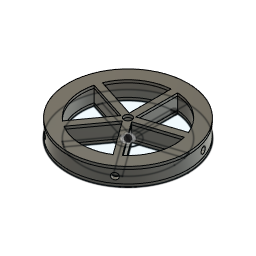
RotarySubAssembly (Autodesk Fusion 360 archive; units mm, degrees)
design "RotarySubFixedTopperV2"
Autodesk Fusion 360 part; units mm, degrees
sketch "Sketch1" plane through (0, 0, 0) normal (0, 1, 0) x (1, 0, 0)
  circle A0 centre (0, 0) radius 3
  circle A1 centre (0, 0) radius 8
  line L0 (0, 0) -> (0, 35)
  line L1 (0, 35) -> (-2.5, 35)
  line L2 (0, 35) -> (2.5, 35)
  line L3 (-2.5, 35) -> (-2.5, 0.0004)
  line L4 (-2.5, 0.0004) -> (2.5, 0.0004)
  line L5 (2.5, 0.0004) -> (2.5, 35)
  line L6 (0.7721, 2.3778) -> (-32.5144, 13.1932)
  line L7 (-34.0595, 8.438) -> (-0.773, -2.3775)
  line L8 (-33.287, 10.8156) -> (-34.0595, 8.438)
  line L9 (-33.287, 10.8156) -> (-32.5144, 13.1932)
  line L10 (-2.0228, 1.4691) -> (-22.595, -26.8461)
  line L11 (-18.5499, -29.7851) -> (2.0223, -1.4698)
  line L12 (-20.5725, -28.3156) -> (-18.5499, -29.7851)
  line L13 (-20.5725, -28.3156) -> (-22.595, -26.8461)
  line L14 (-2.0223, -1.4698) -> (18.5499, -29.7851)
  line L15 (22.595, -26.8461) -> (2.0228, 1.4691)
  line L16 (20.5725, -28.3156) -> (22.595, -26.8461)
  line L17 (20.5725, -28.3156) -> (18.5499, -29.7851)
  line L18 (0.773, -2.3775) -> (34.0595, 8.438)
  line L19 (32.5144, 13.1932) -> (-0.7721, 2.3778)
  line L20 (33.287, 10.8156) -> (32.5144, 13.1932)
  line L21 (33.287, 10.8156) -> (34.0595, 8.438)
  circle A2 centre (0, 0) radius 35
  line L22 (0, 35) -> (0, 45)
  circle A3 centre (0, 0) radius 45
  point P0 (0, 35)
  dimension "d1" = 6
  dimension "d2" = 16
  dimension "d3" = 35
  dimension "d4" = 2.5
  dimension "d6" = 360
  dimension "d7" = 10
  constraint coincident A0.centre A1.centre
  constraint vertical L0
  constraint perpendicular L0 L1
  constraint perpendicular L0 L2
  constraint equal L1 L2
  constraint perpendicular L1 L3
  constraint perpendicular L3 L4
  constraint perpendicular L2 L5
  constraint concentric A0 A2
  constraint coincident P0 L0.end
  constraint tangent L2 A2
  constraint perpendicular L1 L22
  constraint concentric A1 A3
  constraint coincident L22.end A3
  measures "d1" diameter of A0
  measures "d2" diameter of A1
  measures "d3" distance of A0.centre P0
  measures "d4" distance of P0 L1.end
  measures "d7" distance of P0 L22.end
extrude "Extrude1" add sketch "Sketch1" along normal blind 2 contours A0 L15 L18 | A0 A1 L5 L15 L18 L19 | A0 A1 L11 L14 L15 L18 | A0 L5 L19 | A0 L11 L14 | A0 A1 L0 L5 L19 | A1 L14 L15 A2 | A1 L18 L19 A2 | A0 A1 L7 L10 L11 L14 | A0 A1 L0 L3 L6 | A1 L0 L5 A2 | L15 L16 A2 | L18 L21 A2 | A0 L7 L10 | A1 L10 L11 A2 | A0 L3 L6 | A1 L0 L3 A2 | L2 L5 A2 | L19 L20 A2 | L14 L17 A2 | A0 A1 L3 L6 L7 L10 | L11 L12 A2 | L1 L3 A2 | A1 L6 L7 A2 | L10 L13 A2 | L7 L8 A2 | L6 L9 A2 | A3 makes body 1
sketch "Sketch2" plane through (0, 2, 0) normal (0, 1, 0) x (-1, 0, 0)
  arc A0 (-32.4294, -13.1656) -> (-2.5, -34.9106) centre (0, 0) ccw
  line L0 (-32.4294, -13.1656) -> (-2.5, -3.441)
  line L1 (-2.5, -3.441) -> (-2.5, -34.9106)
  arc A1 (2.5, -34.9106) -> (32.4294, -13.1656) centre (0, 0) ccw
  line L2 (2.5, -34.9106) -> (2.5, -3.441)
  line L3 (2.5, -3.441) -> (32.4294, -13.1656)
  line L4 (-22.5425, 26.7738) -> (-4.0451, 1.3143)
  line L5 (-4.0451, 1.3143) -> (-33.9745, -8.4103)
  arc A2 (-22.5425, 26.7738) -> (-33.9745, -8.4103) centre (0, 0) ccw
  arc A3 (33.9745, -8.4103) -> (22.5425, 26.7738) centre (0, 0) ccw
  line L6 (33.9745, -8.4103) -> (4.0451, 1.3143)
  line L7 (4.0451, 1.3143) -> (22.5425, 26.7738)
  arc A4 (18.4974, 29.7127) -> (-18.4974, 29.7127) centre (0, 0) ccw
  line L8 (18.4974, 29.7127) -> (0, 4.2533)
  line L9 (0, 4.2533) -> (-18.4974, 29.7127)
  circle A5 centre (0, 0) radius 3
  circle A6 centre (0, 0) radius 45
  circle A7 centre (0, 0) radius 35
  circle A8 centre (0, 0) radius 45
  line L10 (4.75, -41.9) -> (-4.75, -41.9)
  line L11 (-4.75, -41.9) -> (-4.75, -38.1)
  line L12 (-4.75, -38.1) -> (4.75, -38.1)
  line L13 (4.75, -38.1) -> (4.75, -41.9)
  line L14 (0, -35) -> (0, -38.1)
  line L15 (0, -45) -> (0, -41.9)
  line L16 (41.3171, -8.4303) -> (38.3814, -17.4653)
  line L17 (38.3814, -17.4653) -> (34.7674, -16.2911)
  line L18 (37.7031, -7.256) -> (41.3171, -8.4303)
  line L19 (34.7674, -16.2911) -> (37.7031, -7.256)
  line L20 (20.7854, 36.6898) -> (28.471, 31.1058)
  line L21 (28.471, 31.1058) -> (26.2374, 28.0316)
  line L22 (18.5518, 33.6155) -> (20.7854, 36.6898)
  line L23 (26.2374, 28.0316) -> (18.5518, 33.6155)
  line L24 (-28.471, 31.1058) -> (-20.7854, 36.6898)
  line L25 (-20.7854, 36.6898) -> (-18.5518, 33.6155)
  line L26 (-26.2374, 28.0316) -> (-28.471, 31.1058)
  line L27 (-18.5518, 33.6155) -> (-26.2374, 28.0316)
  line L28 (-38.3814, -17.4653) -> (-41.3171, -8.4303)
  line L29 (-41.3171, -8.4303) -> (-37.7031, -7.256)
  line L30 (-34.7674, -16.2911) -> (-38.3814, -17.4653)
  line L31 (-37.7031, -7.256) -> (-34.7674, -16.2911)
  dimension "d10" = 9.5
  dimension "d11" = 3.8
  dimension "d13" = 360
  constraint horizontal L10
  constraint vertical L11
  constraint horizontal L12
  constraint vertical L13
  constraint coincident A7 L14.start
  constraint vertical L14
  constraint midpoint L12 L14.end
  constraint coincident A6 L15.start
  constraint vertical L15
  constraint midpoint L10 L15.end
  constraint equal L14 L15
  constraint vertical A0.centre L14.end
  measures "d10" distance of L10.start L10.end
  measures "d11" distance of L10.start L12.end
extrude "Extrude2" add sketch "Sketch2" along normal blind 9.5 separate body contours L0 L1 L2 L3 L4 L5 L6 L7 L8 L9 A7 | A6 A8 makes body 2
sketch "Sketch3" plane through (0, 0, -41.9) normal (0, 0, 1) x (1, 0, 0)
  line L0 (-4.75, 2) -> (4.75, 2)
  line L1 (4.75, 2) -> (4.75, 11.5)
  line L2 (4.75, 11.5) -> (-4.75, 11.5)
  line L3 (-4.75, 11.5) -> (-4.75, 2)
  line L4 (-4.75, 11.5) -> (4.75, 2) construction
  line L5 (4.75, 11.5) -> (-4.75, 2) construction
  circle A0 centre (0, 6.75) radius 2.4
  dimension "d16" = 4.8
  constraint coincident L2.end L3.start
  constraint coincident L0.end L1.start
  constraint coincident L1.end L2.start
  constraint coincident L0.start L3.end
  constraint midpoint L5 A0.centre
  measures "d16" diameter of A0
extrude "Extrude3" cut sketch "Sketch3" against normal through all contours A0 bodies 2
pattern_circular "C-Pattern1" count 5 over 360 about axis through (0, 2, 0) along (0, 1, 0) of "Extrude3"
sketch "Sketch4" plane through (0, 11.5, 0) normal (0, 1, 0) x (-1, 0, 0)
  arc A0 (18.4974, 29.7127) -> (-18.4974, 29.7127) centre (0, 0) ccw
  line L0 (18.4974, 29.7127) -> (0, 4.2533)
  line L1 (0, 4.2533) -> (-18.4974, 29.7127)
  arc A1 (2.5, -34.9106) -> (32.4294, -13.1656) centre (0, 0) ccw
  line L2 (2.5, -34.9106) -> (2.5, -3.441)
  line L3 (2.5, -3.441) -> (32.4294, -13.1656)
  arc A2 (-22.5425, 26.7738) -> (-33.9745, -8.4103) centre (0, 0) ccw
  line L4 (-22.5425, 26.7738) -> (-4.0451, 1.3143)
  line L5 (-4.0451, 1.3143) -> (-33.9745, -8.4103)
  arc A3 (-32.4294, -13.1656) -> (-2.5, -34.9106) centre (0, 0) ccw
  line L6 (-32.4294, -13.1656) -> (-2.5, -3.441)
  line L7 (-2.5, -3.441) -> (-2.5, -34.9106)
  line L8 (33.9745, -8.4103) -> (4.0451, 1.3143)
  line L9 (4.0451, 1.3143) -> (22.5425, 26.7738)
  arc A4 (33.9745, -8.4103) -> (22.5425, 26.7738) centre (0, 0) ccw
  line L10 (-4.75, -38.1) -> (4.75, -38.1)
  line L11 (4.75, -38.1) -> (4.75, -41.9)
  line L12 (4.75, -41.9) -> (-4.75, -41.9)
  line L13 (-4.75, -41.9) -> (-4.75, -38.1)
  circle A5 centre (0, 0) radius 3
  line L14 (-20.7854, 36.6898) -> (-18.5518, 33.6155)
  line L15 (-18.5518, 33.6155) -> (-26.2374, 28.0316)
  line L16 (-26.2374, 28.0316) -> (-28.471, 31.1058)
  line L17 (-28.471, 31.1058) -> (-20.7854, 36.6898)
  line L18 (-41.3171, -8.4303) -> (-37.7031, -7.256)
  line L19 (-37.7031, -7.256) -> (-34.7674, -16.2911)
  line L20 (-34.7674, -16.2911) -> (-38.3814, -17.4653)
  line L21 (-38.3814, -17.4653) -> (-41.3171, -8.4303)
  line L22 (28.471, 31.1058) -> (26.2374, 28.0316)
  line L23 (26.2374, 28.0316) -> (18.5518, 33.6155)
  line L24 (18.5518, 33.6155) -> (20.7854, 36.6898)
  line L25 (20.7854, 36.6898) -> (28.471, 31.1058)
  line L26 (38.3814, -17.4653) -> (34.7674, -16.2911)
  line L27 (34.7674, -16.2911) -> (37.7031, -7.256)
  line L28 (37.7031, -7.256) -> (41.3171, -8.4303)
  line L29 (41.3171, -8.4303) -> (38.3814, -17.4653)
  circle A6 centre (0, 0) radius 45
extrude "Extrude4" add sketch "Sketch4" along normal blind 2 separate body contours L10 L11 L12 L13 | L14 L15 L16 L17 | L18 L19 L20 L21 | L22 L23 L24 L25 | L26 L27 L28 L29 | A6 makes body 3
